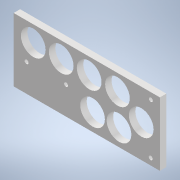
# Autodesk Inventor part: Conectores2
Saved by Autodesk Inventor 2020.3 (Build 243373000, 373)
## iProperties
Created: 2021-04-09
Part Number: Conectores2
Material: Generic
Document SubType Name: Modeling
Designer: juanp
Density: 1 g/cm^3
Appearance: Default
Autodesk Inventor part; units mm, degrees
(part 1 of 2)
ref_plane "YZ Plane" through (0, 0, 0) normal (1, 0, 0) x (0, 1, 0)
ref_plane "XZ Plane" through (0, 0, 0) normal (0, 1, 0) x (-1, 0, 0)
ref_plane "XY Plane" through (0, 0, 0) normal (0, 0, 1) x (1, 0, 0)
sketch "20" plane through (0, 0, 0) normal (0, 0, 1) x (1, 0, 0)
  line L0 (0, 0) -> (106.66, 0)
  line L1 (106.66, 0) -> (106.66, 46.914)
  line L2 (106.66, 46.914) -> (0, 46.914)
  line L3 (0, 46.914) -> (0, 0)
  arc A0 (-5.7307, 23.3678) -> (-5.7307, 23.444) centre (-5.7307, 23.4059) ccw
  line L4 (-5.821, 23.4059) -> (-5.821, 23.4962)
  arc A1 (-5.7829, 23.4962) -> (-5.8591, 23.4962) centre (-5.821, 23.4962) ccw
  arc A2 (-5.8591, 23.4059) -> (-5.7829, 23.4059) centre (-5.821, 23.4059) ccw
  line L5 (-5.821, 23.4962) -> (-5.7307, 23.4962)
  arc A3 (-5.7307, 23.4581) -> (-5.7307, 23.5343) centre (-5.7307, 23.4962) ccw
  arc A4 (-5.821, 23.5343) -> (-5.821, 23.4581) centre (-5.821, 23.4962) ccw
  line L6 (-5.7307, 23.4962) -> (-5.7307, 23.4059)
  arc A5 (-5.7688, 23.4059) -> (-5.6926, 23.4059) centre (-5.7307, 23.4059) ccw
  arc A6 (-5.6926, 23.4962) -> (-5.7688, 23.4962) centre (-5.7307, 23.4962) ccw
  line L7 (-6.4532, 24.9968) -> (-6.4532, 24.4549)
  arc A7 (-6.4913, 24.4549) -> (-6.4151, 24.4549) centre (-6.4532, 24.4549) ccw
  arc A8 (-6.4151, 24.9968) -> (-6.4913, 24.9968) centre (-6.4532, 24.9968) ccw
  arc A9 (-6.8144, 24.0937) -> (-6.4532, 24.4549) centre (-6.8144, 24.4549) ccw
  arc A10 (-6.8144, 24.1318) -> (-6.8144, 24.0556) centre (-6.8144, 24.0937) ccw
  arc A11 (-6.4151, 24.4549) -> (-6.4913, 24.4549) centre (-6.4532, 24.4549) ccw
  line L8 (-6.8144, 24.0937) -> (-6.9047, 24.0937)
  arc A12 (-6.9047, 24.1318) -> (-6.9047, 24.0556) centre (-6.9047, 24.0937) ccw
  arc A13 (-6.8144, 24.0556) -> (-6.8144, 24.1318) centre (-6.8144, 24.0937) ccw
  arc A14 (-6.9047, 24.9968) -> (-6.9047, 24.0937) centre (-6.9047, 24.5453) ccw
  arc A15 (-6.9047, 24.9587) -> (-6.9047, 25.0349) centre (-6.9047, 24.9968) ccw
  arc A16 (-6.9047, 24.0556) -> (-6.9047, 24.1318) centre (-6.9047, 24.0937) ccw
  line L9 (-6.9047, 24.9968) -> (-6.4532, 24.9968)
  arc A17 (-6.4532, 24.9587) -> (-6.4532, 25.0349) centre (-6.4532, 24.9968) ccw
  arc A18 (-6.9047, 25.0349) -> (-6.9047, 24.9587) centre (-6.9047, 24.9968) ccw
  arc A19 (-5.7307, 24.2743) -> (-6.4532, 24.9968) centre (-6.4532, 24.2743) ccw
  arc A20 (-5.7688, 24.2743) -> (-5.6926, 24.2743) centre (-5.7307, 24.2743) ccw
  arc A21 (-6.4532, 25.0349) -> (-6.4532, 24.9587) centre (-6.4532, 24.9968) ccw
  line L10 (-6.9951, 25.6568) -> (-7.3563, 26.1084)
  arc A22 (-7.3265, 26.1322) -> (-7.3861, 26.0846) centre (-7.3563, 26.1084) ccw
  arc A23 (-7.0248, 25.633) -> (-6.9653, 25.6806) centre (-6.9951, 25.6568) ccw
  line L11 (-7.3563, 26.1084) -> (-5.7307, 26.1084)
  arc A24 (-5.7307, 26.0703) -> (-5.7307, 26.1465) centre (-5.7307, 26.1084) ccw
  arc A25 (-7.3563, 26.1465) -> (-7.3563, 26.0703) centre (-7.3563, 26.1084) ccw
  line L12 (-5.7307, 25.6568) -> (-5.7307, 26.5599)
  arc A26 (-5.6926, 26.5599) -> (-5.7688, 26.5599) centre (-5.7307, 26.5599) ccw
  arc A27 (-5.7688, 25.6568) -> (-5.6926, 25.6568) centre (-5.7307, 25.6568) ccw
  line L13 (106.66, 46.914) -> (106.66, 51.48)
  arc A28 (106.6925, 51.48) -> (106.6275, 51.48) centre (106.66, 51.48) ccw
  arc A29 (106.6275, 46.914) -> (106.6925, 46.914) centre (106.66, 46.914) ccw
  line L14 (0, 46.914) -> (0, 51.48)
  arc A30 (0.0325, 51.48) -> (-0.0325, 51.48) centre (0, 51.48) ccw
  arc A31 (-0.0325, 46.914) -> (0.0325, 46.914) centre (0, 46.914) ccw
  line L15 (106.595, 49.53) -> (0.065, 49.53)
  arc A32 (0.065, 49.5625) -> (0.065, 49.4975) centre (0.065, 49.53) ccw
  arc A33 (106.595, 49.4975) -> (106.595, 49.5625) centre (106.595, 49.53) ccw
  line L16 (106.595, 49.53) -> (104.06, 49.8492)
  arc A34 (104.0641, 49.8815) -> (104.0559, 49.817) centre (104.06, 49.8493) ccw
  arc A35 (106.5909, 49.4978) -> (106.5991, 49.5622) centre (106.595, 49.53) ccw
  line L17 (104.06, 49.8492) -> (104.06, 49.2108)
  arc A36 (104.0275, 49.2108) -> (104.0925, 49.2108) centre (104.06, 49.2108) ccw
  arc A37 (104.0925, 49.8492) -> (104.0275, 49.8492) centre (104.06, 49.8492) ccw
  line L18 (104.06, 49.2108) -> (106.595, 49.53)
  arc A38 (106.5991, 49.4978) -> (106.5909, 49.5622) centre (106.595, 49.53) ccw
  arc A39 (104.0559, 49.243) -> (104.0641, 49.1785) centre (104.06, 49.2107) ccw
  line L19 (106.595, 49.53) -> (104.06, 49.66)
  arc A40 (104.0617, 49.6925) -> (104.0583, 49.6275) centre (104.06, 49.66) ccw
  arc A41 (106.5933, 49.4975) -> (106.5967, 49.5625) centre (106.595, 49.53) ccw
  line L20 (104.06, 49.4) -> (106.595, 49.53)
  arc A42 (106.5967, 49.4975) -> (106.5933, 49.5625) centre (106.595, 49.53) ccw
  arc A43 (104.0583, 49.4325) -> (104.0617, 49.3675) centre (104.06, 49.4) ccw
  line L21 (106.595, 49.53) -> (104.06, 49.79)
  arc A44 (104.0633, 49.8223) -> (104.0567, 49.7577) centre (104.06, 49.79) ccw
  arc A45 (106.5917, 49.4977) -> (106.5983, 49.5623) centre (106.595, 49.53) ccw
  line L22 (104.06, 49.27) -> (106.595, 49.53)
  arc A46 (106.5983, 49.4977) -> (106.5917, 49.5623) centre (106.595, 49.53) ccw
  arc A47 (104.0567, 49.3023) -> (104.0633, 49.2377) centre (104.06, 49.27) ccw
  line L23 (0.065, 49.53) -> (2.6, 49.8492)
  arc A48 (2.6041, 49.817) -> (2.5959, 49.8815) centre (2.6, 49.8493) ccw
  arc A49 (0.0609, 49.5622) -> (0.0691, 49.4978) centre (0.065, 49.53) ccw
  line L24 (2.6, 49.8492) -> (2.6, 49.2108)
  arc A50 (2.5675, 49.2108) -> (2.6325, 49.2108) centre (2.6, 49.2108) ccw
  arc A51 (2.6325, 49.8492) -> (2.5675, 49.8492) centre (2.6, 49.8492) ccw
  line L25 (2.6, 49.2108) -> (0.065, 49.53)
  arc A52 (0.0691, 49.5622) -> (0.0609, 49.4978) centre (0.065, 49.53) ccw
  arc A53 (2.5959, 49.1785) -> (2.6041, 49.243) centre (2.6, 49.2107) ccw
  line L26 (0.065, 49.53) -> (2.6, 49.66)
  arc A54 (2.6017, 49.6275) -> (2.5983, 49.6925) centre (2.6, 49.66) ccw
  arc A55 (0.0633, 49.5625) -> (0.0667, 49.4975) centre (0.065, 49.53) ccw
  line L27 (2.6, 49.4) -> (0.065, 49.53)
  arc A56 (0.0667, 49.5625) -> (0.0633, 49.4975) centre (0.065, 49.53) ccw
  arc A57 (2.5983, 49.3675) -> (2.6017, 49.4325) centre (2.6, 49.4) ccw
  line L28 (0.065, 49.53) -> (2.6, 49.79)
  arc A58 (2.6033, 49.7577) -> (2.5967, 49.8223) centre (2.6, 49.79) ccw
  arc A59 (0.0617, 49.5623) -> (0.0683, 49.4977) centre (0.065, 49.53) ccw
  line L29 (2.6, 49.27) -> (0.065, 49.53)
  arc A60 (0.0683, 49.5623) -> (0.0617, 49.4977) centre (0.065, 49.53) ccw
  arc A61 (2.5967, 49.2377) -> (2.6033, 49.3023) centre (2.6, 49.27) ccw
  line L30 (49.5056, 51.4451) -> (49.9571, 51.8063)
  arc A62 (49.9809, 51.7765) -> (49.9333, 51.8361) centre (49.9571, 51.8063) ccw
  arc A63 (49.4818, 51.4748) -> (49.5294, 51.4153) centre (49.5056, 51.4451) ccw
  line L31 (49.9571, 51.8063) -> (49.9571, 50.1807)
  arc A64 (49.919, 50.1807) -> (49.9952, 50.1807) centre (49.9571, 50.1807) ccw
  arc A65 (49.9952, 51.8063) -> (49.919, 51.8063) centre (49.9571, 51.8063) ccw
  line L32 (49.5056, 50.1807) -> (50.4087, 50.1807)
  arc A66 (50.4087, 50.1426) -> (50.4087, 50.2188) centre (50.4087, 50.1807) ccw
  arc A67 (49.5056, 50.2188) -> (49.5056, 50.1426) centre (49.5056, 50.1807) ccw
  arc A68 (51.2042, 51.5805) -> (51.0687, 50.9935) centre (52.4081, 50.9934) ccw
  arc A69 (51.2384, 51.5638) -> (51.1699, 51.5972) centre (51.2042, 51.5805) ccw
  arc A70 (51.0306, 50.9935) -> (51.1068, 50.9935) centre (51.0687, 50.9935) ccw
  arc A71 (51.5203, 51.8063) -> (51.2042, 51.5805) centre (51.5203, 51.4722) ccw
  arc A72 (51.5203, 51.7682) -> (51.5203, 51.8444) centre (51.5203, 51.8063) ccw
  arc A73 (51.1681, 51.5929) -> (51.2402, 51.5682) centre (51.2042, 51.5806) ccw
  arc A74 (51.8364, 51.5805) -> (51.5203, 51.8063) centre (51.5203, 51.4722) ccw
  arc A75 (51.8003, 51.5682) -> (51.8724, 51.5929) centre (51.8363, 51.5806) ccw
  arc A76 (51.5203, 51.8444) -> (51.5203, 51.7682) centre (51.5203, 51.8063) ccw
  arc A77 (51.9718, 50.9935) -> (51.8364, 51.5805) centre (50.6324, 50.9937) ccw
  arc A78 (51.9337, 50.9935) -> (52.0099, 50.9935) centre (51.9718, 50.9935) ccw
  arc A79 (51.8706, 51.5972) -> (51.8021, 51.5638) centre (51.8364, 51.5805) ccw
  arc A80 (51.0687, 50.9935) -> (51.2042, 50.4065) centre (52.4081, 50.9936) ccw
  arc A81 (51.1068, 50.9935) -> (51.0306, 50.9935) centre (51.0687, 50.9935) ccw
  arc A82 (51.1699, 50.3898) -> (51.2384, 50.4232) centre (51.2042, 50.4065) ccw
  arc A83 (51.2042, 50.4065) -> (51.5203, 50.1807) centre (51.5203, 50.5148) ccw
  arc A84 (51.2402, 50.4188) -> (51.1681, 50.3941) centre (51.2042, 50.4065) ccw
  arc A85 (51.5203, 50.1426) -> (51.5203, 50.2188) centre (51.5203, 50.1807) ccw
  arc A86 (51.8364, 50.4065) -> (51.9718, 50.9935) centre (50.6324, 50.9933) ccw
  arc A87 (51.8021, 50.4232) -> (51.8706, 50.3898) centre (51.8364, 50.4065) ccw
  arc A88 (52.0099, 50.9935) -> (51.9337, 50.9935) centre (51.9718, 50.9935) ccw
  arc A89 (51.5203, 50.1807) -> (51.8364, 50.4065) centre (51.5203, 50.5148) ccw
  arc A90 (51.5203, 50.2188) -> (51.5203, 50.1426) centre (51.5203, 50.1807) ccw
  arc A91 (51.8724, 50.3941) -> (51.8003, 50.4188) centre (51.8363, 50.4065) ccw
  line L33 (51.159, 50.5419) -> (51.8815, 51.4451)
  arc A92 (51.9113, 51.4213) -> (51.8518, 51.4689) centre (51.8816, 51.4451) ccw
  arc A93 (51.1293, 50.5657) -> (51.1888, 50.5181) centre (51.1591, 50.5419) ccw
  line L34 (52.6318, 51.0838) -> (53.1737, 51.0838)
  arc A94 (53.1737, 51.0457) -> (53.1737, 51.1219) centre (53.1737, 51.0838) ccw
  arc A95 (52.6318, 51.1219) -> (52.6318, 51.0457) centre (52.6318, 51.0838) ccw
  arc A96 (53.5349, 50.7226) -> (53.1737, 51.0838) centre (53.1737, 50.7226) ccw
  arc A97 (53.4968, 50.7226) -> (53.573, 50.7226) centre (53.5349, 50.7226) ccw
  arc A98 (53.1737, 51.1219) -> (53.1737, 51.0457) centre (53.1737, 51.0838) ccw
  line L35 (53.5349, 50.7226) -> (53.5349, 50.6323)
  arc A99 (53.4968, 50.6323) -> (53.573, 50.6323) centre (53.5349, 50.6323) ccw
  arc A100 (53.573, 50.7226) -> (53.4968, 50.7226) centre (53.5349, 50.7226) ccw
  arc A101 (52.6318, 50.6323) -> (53.5349, 50.6323) centre (53.0833, 50.6323) ccw
  arc A102 (52.6699, 50.6323) -> (52.5937, 50.6323) centre (52.6318, 50.6323) ccw
  arc A103 (53.573, 50.6323) -> (53.4968, 50.6323) centre (53.5349, 50.6323) ccw
  line L36 (52.6318, 50.6323) -> (52.6318, 51.0838)
  arc A104 (52.6699, 51.0838) -> (52.5937, 51.0838) centre (52.6318, 51.0838) ccw
  arc A105 (56.3452, 50.6323) -> (56.4214, 50.6323) centre (56.3833, 50.6323) ccw
  arc A106 (52.5937, 50.6323) -> (52.6699, 50.6323) centre (52.6318, 50.6323) ccw
  arc A107 (53.3543, 51.8063) -> (52.6318, 51.0838) centre (53.3543, 51.0838) ccw
  arc A108 (53.3543, 51.7682) -> (53.3543, 51.8444) centre (53.3543, 51.8063) ccw
  arc A109 (52.5937, 51.0838) -> (52.6699, 51.0838) centre (52.6318, 51.0838) ccw
  line L37 (54.1324, 50.1807) -> (54.1324, 50.271)
  arc A110 (54.1705, 50.271) -> (54.0943, 50.271) centre (54.1324, 50.271) ccw
  arc A111 (54.0943, 50.1807) -> (54.1705, 50.1807) centre (54.1324, 50.1807) ccw
  line L38 (54.1324, 50.271) -> (54.2227, 50.271)
  arc A112 (54.2227, 50.2329) -> (54.2227, 50.3091) centre (54.2227, 50.271) ccw
  arc A113 (54.1324, 50.3091) -> (54.1324, 50.2329) centre (54.1324, 50.271) ccw
  line L39 (54.2227, 50.271) -> (54.2227, 50.1807)
  arc A114 (54.1846, 50.1807) -> (54.2608, 50.1807) centre (54.2227, 50.1807) ccw
  arc A115 (54.2608, 50.271) -> (54.1846, 50.271) centre (54.2227, 50.271) ccw
  line L40 (54.2227, 50.1807) -> (54.1324, 50.1807)
  arc A116 (54.1324, 50.2188) -> (54.1324, 50.1426) centre (54.1324, 50.1807) ccw
  arc A117 (54.2227, 50.1426) -> (54.2227, 50.2188) centre (54.2227, 50.1807) ccw
  arc A118 (55.3621, 51.0457) -> (55.3621, 51.1219) centre (55.3621, 51.0838) ccw
  arc A119 (54.8202, 51.1219) -> (54.8202, 51.0457) centre (54.8202, 51.0838) ccw
  arc A120 (55.7233, 50.7226) -> (55.3621, 51.0838) centre (55.3621, 50.7226) ccw
  arc A121 (55.6852, 50.7226) -> (55.7614, 50.7226) centre (55.7233, 50.7226) ccw
  arc A122 (55.3621, 51.1219) -> (55.3621, 51.0457) centre (55.3621, 51.0838) ccw
  line L41 (55.7233, 50.7226) -> (55.7233, 50.6323)
  arc A123 (55.6852, 50.6323) -> (55.7614, 50.6323) centre (55.7233, 50.6323) ccw
  arc A124 (55.7614, 50.7226) -> (55.6852, 50.7226) centre (55.7233, 50.7226) ccw
  arc A125 (54.8202, 50.6323) -> (55.7233, 50.6323) centre (55.2717, 50.6323) ccw
  arc A126 (54.8583, 50.6323) -> (54.7821, 50.6323) centre (54.8202, 50.6323) ccw
  arc A127 (55.7614, 50.6323) -> (55.6852, 50.6323) centre (55.7233, 50.6323) ccw
  line L42 (54.8202, 50.6323) -> (54.8202, 51.0838)
  arc A128 (54.8583, 51.0838) -> (54.7821, 51.0838) centre (54.8202, 51.0838) ccw
  arc A129 (54.7821, 50.6323) -> (54.8583, 50.6323) centre (54.8202, 50.6323) ccw
  arc A130 (55.5427, 51.8063) -> (54.8202, 51.0838) centre (55.5427, 51.0838) ccw
  arc A131 (55.5427, 51.7682) -> (55.5427, 51.8444) centre (55.5427, 51.8063) ccw
  arc A132 (54.7821, 51.0838) -> (54.8583, 51.0838) centre (54.8202, 51.0838) ccw
  line L43 (56.3833, 51.0838) -> (56.9252, 51.0838)
  arc A133 (56.9252, 51.0457) -> (56.9252, 51.1219) centre (56.9252, 51.0838) ccw
  arc A134 (56.3833, 51.1219) -> (56.3833, 51.0457) centre (56.3833, 51.0838) ccw
  arc A135 (57.2864, 50.7226) -> (56.9252, 51.0838) centre (56.9252, 50.7226) ccw
  arc A136 (57.2483, 50.7226) -> (57.3245, 50.7226) centre (57.2864, 50.7226) ccw
  arc A137 (56.9252, 51.1219) -> (56.9252, 51.0457) centre (56.9252, 51.0838) ccw
  line L44 (57.2864, 50.7226) -> (57.2864, 50.6323)
  arc A138 (57.2483, 50.6323) -> (57.3245, 50.6323) centre (57.2864, 50.6323) ccw
  arc A139 (57.3245, 50.7226) -> (57.2483, 50.7226) centre (57.2864, 50.7226) ccw
  arc A140 (56.3833, 50.6323) -> (57.2864, 50.6323) centre (56.8349, 50.6323) ccw
  arc A141 (56.4214, 50.6323) -> (56.3452, 50.6323) centre (56.3833, 50.6323) ccw
  arc A142 (57.3245, 50.6323) -> (57.2483, 50.6323) centre (57.2864, 50.6323) ccw
  line L45 (56.3833, 50.6323) -> (56.3833, 51.0838)
  arc A143 (56.4214, 51.0838) -> (56.3452, 51.0838) centre (56.3833, 51.0838) ccw
  line L46 (2.54, 46.914) -> (-7.03, 46.914)
  arc A144 (-7.03, 46.9465) -> (-7.03, 46.8815) centre (-7.03, 46.914) ccw
  arc A145 (2.54, 46.8815) -> (2.54, 46.9465) centre (2.54, 46.914) ccw
  line L47 (2.54, 0) -> (-7.03, 0)
  arc A146 (-7.03, 0.0325) -> (-7.03, -0.0325) centre (-7.03, 0) ccw
  arc A147 (2.54, -0.0325) -> (2.54, 0.0325) centre (2.54, 0) ccw
  line L48 (-5.08, 46.849) -> (-5.08, 0.065)
  arc A148 (-5.1125, 0.065) -> (-5.0475, 0.065) centre (-5.08, 0.065) ccw
  arc A149 (-5.0475, 46.849) -> (-5.1125, 46.849) centre (-5.08, 46.849) ccw
  line L49 (-5.08, 46.849) -> (-5.3992, 44.314)
  arc A150 (-5.4315, 44.3181) -> (-5.367, 44.3099) centre (-5.3993, 44.314) ccw
  arc A151 (-5.0478, 46.8449) -> (-5.1122, 46.8531) centre (-5.08, 46.849) ccw
  line L50 (-5.3992, 44.314) -> (-4.7608, 44.314)
  arc A152 (-4.7608, 44.2815) -> (-4.7608, 44.3465) centre (-4.7608, 44.314) ccw
  arc A153 (-5.3992, 44.3465) -> (-5.3992, 44.2815) centre (-5.3992, 44.314) ccw
  line L51 (-4.7608, 44.314) -> (-5.08, 46.849)
  arc A154 (-5.0478, 46.8531) -> (-5.1122, 46.8449) centre (-5.08, 46.849) ccw
  arc A155 (-4.793, 44.3099) -> (-4.7285, 44.3181) centre (-4.7607, 44.314) ccw
  line L52 (-5.08, 46.849) -> (-5.21, 44.314)
  arc A156 (-5.2425, 44.3157) -> (-5.1775, 44.3123) centre (-5.21, 44.314) ccw
  arc A157 (-5.0475, 46.8473) -> (-5.1125, 46.8507) centre (-5.08, 46.849) ccw
  line L53 (-4.95, 44.314) -> (-5.08, 46.849)
  arc A158 (-5.0475, 46.8507) -> (-5.1125, 46.8473) centre (-5.08, 46.849) ccw
  arc A159 (-4.9825, 44.3123) -> (-4.9175, 44.3157) centre (-4.95, 44.314) ccw
  line L54 (-5.08, 46.849) -> (-5.34, 44.314)
  arc A160 (-5.3723, 44.3173) -> (-5.3077, 44.3107) centre (-5.34, 44.314) ccw
  arc A161 (-5.0477, 46.8457) -> (-5.1123, 46.8523) centre (-5.08, 46.849) ccw
  line L55 (-4.82, 44.314) -> (-5.08, 46.849)
  arc A162 (-5.0477, 46.8523) -> (-5.1123, 46.8457) centre (-5.08, 46.849) ccw
  arc A163 (-4.8523, 44.3107) -> (-4.7877, 44.3173) centre (-4.82, 44.314) ccw
  line L56 (-5.08, 0.065) -> (-5.3992, 2.6)
  arc A164 (-5.367, 2.6041) -> (-5.4315, 2.5959) centre (-5.3993, 2.6) ccw
  arc A165 (-5.1122, 0.0609) -> (-5.0478, 0.0691) centre (-5.08, 0.065) ccw
  line L57 (-5.3992, 2.6) -> (-4.7608, 2.6)
  arc A166 (-4.7608, 2.5675) -> (-4.7608, 2.6325) centre (-4.7608, 2.6) ccw
  arc A167 (-5.3992, 2.6325) -> (-5.3992, 2.5675) centre (-5.3992, 2.6) ccw
  line L58 (-4.7608, 2.6) -> (-5.08, 0.065)
  arc A168 (-5.1122, 0.0691) -> (-5.0478, 0.0609) centre (-5.08, 0.065) ccw
  arc A169 (-4.7285, 2.5959) -> (-4.793, 2.6041) centre (-4.7607, 2.6) ccw
  line L59 (-5.08, 0.065) -> (-5.21, 2.6)
  arc A170 (-5.1775, 2.6017) -> (-5.2425, 2.5983) centre (-5.21, 2.6) ccw
  arc A171 (-5.1125, 0.0633) -> (-5.0475, 0.0667) centre (-5.08, 0.065) ccw
  line L60 (-4.95, 2.6) -> (-5.08, 0.065)
  arc A172 (-5.1125, 0.0667) -> (-5.0475, 0.0633) centre (-5.08, 0.065) ccw
  arc A173 (-4.9175, 2.5983) -> (-4.9825, 2.6017) centre (-4.95, 2.6) ccw
  line L61 (-5.08, 0.065) -> (-5.34, 2.6)
  arc A174 (-5.3077, 2.6033) -> (-5.3723, 2.5967) centre (-5.34, 2.6) ccw
  arc A175 (-5.1123, 0.0617) -> (-5.0477, 0.0683) centre (-5.08, 0.065) ccw
  line L62 (-4.82, 2.6) -> (-5.08, 0.065)
  arc A176 (-5.1123, 0.0683) -> (-5.0477, 0.0617) centre (-5.08, 0.065) ccw
  arc A177 (-4.7877, 2.5967) -> (-4.8523, 2.6033) centre (-4.82, 2.6) ccw
  line L63 (-7.3563, 20.7034) -> (-6.0919, 20.3422)
  arc A178 (-6.1024, 20.3056) -> (-6.0815, 20.3788) centre (-6.092, 20.3422) ccw
  arc A179 (-7.3458, 20.7401) -> (-7.3668, 20.6668) centre (-7.3563, 20.7035) ccw
  line L64 (-6.0919, 20.3422) -> (-6.0919, 21.2453)
  arc A180 (-6.0538, 21.2453) -> (-6.13, 21.2453) centre (-6.0919, 21.2453) ccw
  arc A181 (-6.13, 20.3422) -> (-6.0538, 20.3422) centre (-6.0919, 20.3422) ccw
  line L65 (-6.4532, 20.9744) -> (-5.7307, 20.9744)
  arc A182 (-5.7307, 20.9363) -> (-5.7307, 21.0125) centre (-5.7307, 20.9744) ccw
  arc A183 (-6.4532, 21.0125) -> (-6.4532, 20.9363) centre (-6.4532, 20.9744) ccw
  line L66 (-6.6338, 21.9053) -> (-6.6338, 22.4472)
  arc A184 (-6.5957, 22.4472) -> (-6.6719, 22.4472) centre (-6.6338, 22.4472) ccw
  arc A185 (-6.6719, 21.9053) -> (-6.5957, 21.9053) centre (-6.6338, 21.9053) ccw
  arc A186 (-6.2726, 22.8084) -> (-6.6338, 22.4472) centre (-6.2726, 22.4472) ccw
  arc A187 (-6.2726, 22.7703) -> (-6.2726, 22.8465) centre (-6.2726, 22.8084) ccw
  arc A188 (-6.6719, 22.4472) -> (-6.5957, 22.4472) centre (-6.6338, 22.4472) ccw
  line L67 (-6.2726, 22.8084) -> (-6.1823, 22.8084)
  arc A189 (-6.1823, 22.7703) -> (-6.1823, 22.8465) centre (-6.1823, 22.8084) ccw
  arc A190 (-6.2726, 22.8465) -> (-6.2726, 22.7703) centre (-6.2726, 22.8084) ccw
  arc A191 (-6.1823, 21.9053) -> (-6.1823, 22.8084) centre (-6.1823, 22.3569) ccw
  arc A192 (-6.1823, 21.9434) -> (-6.1823, 21.8672) centre (-6.1823, 21.9053) ccw
  arc A193 (-6.1823, 22.8465) -> (-6.1823, 22.7703) centre (-6.1823, 22.8084) ccw
  line L68 (-6.1823, 21.9053) -> (-6.6338, 21.9053)
  arc A194 (-6.6338, 21.9434) -> (-6.6338, 21.8672) centre (-6.6338, 21.9053) ccw
  arc A195 (-6.1823, 21.8672) -> (-6.1823, 21.9434) centre (-6.1823, 21.9053) ccw
  arc A196 (-7.3563, 22.6278) -> (-6.6338, 21.9053) centre (-6.6338, 22.6278) ccw
  arc A197 (-7.3182, 22.6278) -> (-7.3944, 22.6278) centre (-7.3563, 22.6278) ccw
  arc A198 (-6.6338, 21.8672) -> (-6.6338, 21.9434) centre (-6.6338, 21.9053) ccw
  line L69 (-5.7307, 23.4059) -> (-5.821, 23.4059)
  arc A199 (-5.821, 23.444) -> (-5.821, 23.3678) centre (-5.821, 23.4059) ccw
  arc A200 (57.1058, 51.8063) -> (56.3833, 51.0838) centre (57.1058, 51.0838) ccw
  arc A201 (57.1058, 51.7682) -> (57.1058, 51.8444) centre (57.1058, 51.8063) ccw
  arc A202 (56.3452, 51.0838) -> (56.4214, 51.0838) centre (56.3833, 51.0838) ccw
  circle A203 centre (6.998, 20.3594) radius 1.51
  circle A204 centre (37.3779, 20.3594) radius 1.51
  circle A205 centre (102.615, 42.9184) radius 1.51
  circle A206 centre (102.502, 4.0549) radius 1.51
  line L70 (54.8202, 51.0838) -> (55.3621, 51.0838)
  constraints: 501 point on circle, 207 centre point, 142 end point, 56 point on line
sketch "21" plane through (0, 0, 0) normal (0, 0, 1) x (1, 0, 0)
  line L0 (56.8302, 12.0686) -> (57.1435, 12.0686)
  line L1 (2.5931, 11.0351) -> (22.5931, 11.0351)
  arc A0 (22.5931, 10.9843) -> (22.5931, 11.0859) centre (22.5931, 11.0351) ccw
  arc A1 (2.5931, 11.0859) -> (2.5931, 10.9843) centre (2.5931, 11.0351) ccw
  line L2 (22.5931, 11.0351) -> (22.5931, 2.6351)
  arc A2 (22.5423, 2.6351) -> (22.6439, 2.6351) centre (22.5931, 2.6351) ccw
  arc A3 (22.6439, 11.0351) -> (22.5423, 11.0351) centre (22.5931, 11.0351) ccw
  line L3 (22.5931, 2.6351) -> (18.5311, 2.6351)
  arc A4 (18.5311, 2.6859) -> (18.5311, 2.5843) centre (18.5311, 2.6351) ccw
  arc A5 (22.5931, 2.5843) -> (22.5931, 2.6859) centre (22.5931, 2.6351) ccw
  line L4 (18.5311, 2.6351) -> (18.5311, 2.9351)
  arc A6 (18.5819, 2.9351) -> (18.4803, 2.9351) centre (18.5311, 2.9351) ccw
  arc A7 (18.4803, 2.6351) -> (18.5819, 2.6351) centre (18.5311, 2.6351) ccw
  line L5 (18.5311, 2.9351) -> (17.0521, 2.9351)
  arc A8 (17.0521, 2.9859) -> (17.0521, 2.8843) centre (17.0521, 2.9351) ccw
  arc A9 (18.5311, 2.8843) -> (18.5311, 2.9859) centre (18.5311, 2.9351) ccw
  line L6 (17.0521, 2.9351) -> (17.0521, 2.6351)
  arc A10 (17.0013, 2.6351) -> (17.1029, 2.6351) centre (17.0521, 2.6351) ccw
  arc A11 (17.1029, 2.9351) -> (17.0013, 2.9351) centre (17.0521, 2.9351) ccw
  line L7 (17.0521, 2.6351) -> (14.4761, 2.6351)
  arc A12 (14.4761, 2.6859) -> (14.4761, 2.5843) centre (14.4761, 2.6351) ccw
  arc A13 (17.0521, 2.5843) -> (17.0521, 2.6859) centre (17.0521, 2.6351) ccw
  line L8 (14.4761, 2.6351) -> (14.4761, 4.1851)
  arc A14 (14.5269, 4.1851) -> (14.4253, 4.1851) centre (14.4761, 4.1851) ccw
  arc A15 (14.4253, 2.6351) -> (14.5269, 2.6351) centre (14.4761, 2.6351) ccw
  line L9 (14.4761, 4.1851) -> (10.7101, 4.1851)
  arc A16 (10.7101, 4.2359) -> (10.7101, 4.1343) centre (10.7101, 4.1851) ccw
  arc A17 (14.4761, 4.1343) -> (14.4761, 4.2359) centre (14.4761, 4.1851) ccw
  line L10 (10.7101, 4.1851) -> (10.7101, 2.6351)
  arc A18 (10.6593, 2.6351) -> (10.7609, 2.6351) centre (10.7101, 2.6351) ccw
  arc A19 (10.7609, 4.1851) -> (10.6593, 4.1851) centre (10.7101, 4.1851) ccw
  line L11 (14.4761, 2.6351) -> (10.7101, 2.6351)
  arc A20 (10.7101, 2.6859) -> (10.7101, 2.5843) centre (10.7101, 2.6351) ccw
  arc A21 (76.2324, 34.6718) -> (76.2324, 34.6337) centre (76.2324, 34.6527) ccw
  arc A22 (76.2324, 35.1939) -> (76.2324, 35.1558) centre (76.2324, 35.1748) ccw
  line L12 (75.9714, 35.5925) -> (76.2847, 35.5925)
  arc A23 (76.2847, 35.5735) -> (76.2847, 35.6116) centre (76.2847, 35.5926) ccw
  arc A24 (75.9714, 35.6116) -> (75.9714, 35.5735) centre (75.9714, 35.5926) ccw
  arc A25 (76.2847, 35.1748) -> (76.2847, 35.5925) centre (76.2847, 35.3837) ccw
  arc A26 (76.2847, 35.1939) -> (76.2847, 35.1558) centre (76.2847, 35.1748) ccw
  arc A27 (76.2847, 35.6116) -> (76.2847, 35.5735) centre (76.2847, 35.5926) ccw
  line L13 (76.2847, 35.1748) -> (76.0758, 35.1748)
  arc A28 (76.0758, 35.1939) -> (76.0758, 35.1558) centre (76.0758, 35.1748) ccw
  arc A29 (75.9714, 34.6718) -> (75.9714, 34.6337) centre (75.9714, 34.6527) ccw
  arc A30 (76.9333, 27.6146) -> (76.9333, 43.6146) centre (76.9333, 35.6146) ccw
  arc A31 (76.9333, 43.6146) -> (76.9333, 27.6146) centre (76.9333, 35.6146) ccw
  arc A32 (76.9333, 29.0954) -> (76.9333, 42.1338) centre (76.9333, 35.6146) ccw
  arc A33 (76.9333, 42.1338) -> (76.9333, 29.0954) centre (76.9333, 35.6146) ccw
  arc A34 (76.9333, 26.1146) -> (76.9333, 45.1146) centre (76.9333, 35.6146) ccw
  arc A35 (76.9333, 45.1146) -> (76.9333, 26.1146) centre (76.9333, 35.6146) ccw
  arc A36 (2.6439, 11.0351) -> (2.5423, 11.0351) centre (2.5931, 11.0351) ccw
  arc A37 (58.7921, 5.5907) -> (56.7921, 5.5907) centre (57.7921, 5.5907) ccw
  arc A38 (58.7604, 5.5907) -> (58.8239, 5.5907) centre (58.7922, 5.5907) ccw
  arc A39 (56.7604, 5.5907) -> (56.8239, 5.5907) centre (56.7921, 5.5907) ccw
  line L14 (62.8302, 11.8597) -> (63.0913, 12.0686)
  arc A40 (63.1032, 12.0537) -> (63.0794, 12.0834) centre (63.0913, 12.0686) ccw
  arc A41 (62.8183, 11.8746) -> (62.8421, 11.8448) centre (62.8302, 11.8597) ccw
  line L15 (63.0913, 12.0686) -> (63.0913, 11.1288)
  arc A42 (63.0722, 11.1288) -> (63.1103, 11.1288) centre (63.0913, 11.1288) ccw
  arc A43 (63.1103, 12.0686) -> (63.0722, 12.0686) centre (63.0913, 12.0686) ccw
  line L16 (62.8302, 11.1288) -> (63.3523, 11.1288)
  arc A44 (63.3523, 11.1097) -> (63.3523, 11.1478) centre (63.3523, 11.1288) ccw
  arc A45 (62.8302, 11.1478) -> (62.8302, 11.1097) centre (62.8302, 11.1288) ccw
  arc A46 (60.3523, 16.8336) -> (60.1174, 17.0686) centre (60.1173, 16.8336) ccw
  arc A47 (60.3333, 16.8336) -> (60.3714, 16.8336) centre (60.3524, 16.8336) ccw
  arc A48 (60.1174, 17.0876) -> (60.1174, 17.0495) centre (60.1174, 17.0686) ccw
  arc A49 (60.1174, 17.0686) -> (59.8302, 16.8597) centre (60.1174, 16.7667) ccw
  arc A50 (60.1174, 17.0495) -> (60.1174, 17.0876) centre (60.1174, 17.0686) ccw
  arc A51 (59.8121, 16.8656) -> (59.8483, 16.8538) centre (59.8302, 16.8597) ccw
  arc A52 (60.274, 16.6509) -> (60.3523, 16.8336) centre (60.0999, 16.8336) ccw
  arc A53 (60.2609, 16.6647) -> (60.2871, 16.6371) centre (60.274, 16.6509) ccw
  arc A54 (60.3714, 16.8336) -> (60.3333, 16.8336) centre (60.3524, 16.8336) ccw
  line L17 (60.274, 16.6509) -> (59.8302, 16.1288)
  arc A55 (59.8157, 16.1411) -> (59.8447, 16.1164) centre (59.8302, 16.1288) ccw
  arc A56 (60.2885, 16.6385) -> (60.2595, 16.6632) centre (60.274, 16.6508) ccw
  line L18 (59.8302, 16.1288) -> (60.3523, 16.1288)
  arc A57 (60.3523, 16.1097) -> (60.3523, 16.1478) centre (60.3523, 16.1288) ccw
  arc A58 (59.8302, 16.1478) -> (59.8302, 16.1097) centre (59.8302, 16.1288) ccw
  line L19 (56.8302, 11.1288) -> (57.0913, 11.1288)
  arc A59 (57.0913, 11.1097) -> (57.0913, 11.1478) centre (57.0913, 11.1288) ccw
  arc A60 (56.8302, 11.1478) -> (56.8302, 11.1097) centre (56.8302, 11.1288) ccw
  arc A61 (57.0913, 11.1288) -> (57.0913, 11.6509) centre (57.0913, 11.3898) ccw
  arc A62 (57.0913, 11.1478) -> (57.0913, 11.1097) centre (57.0913, 11.1288) ccw
  arc A63 (57.0913, 11.6699) -> (57.0913, 11.6318) centre (57.0913, 11.6509) ccw
  arc A64 (80.6119, 16.6647) -> (80.6381, 16.6371) centre (80.625, 16.6509) ccw
  arc A65 (57.1435, 12.0495) -> (57.1435, 12.0876) centre (57.1435, 12.0686) ccw
  arc A66 (56.8302, 12.0876) -> (56.8302, 12.0495) centre (56.8302, 12.0686) ccw
  arc A67 (57.1435, 11.6509) -> (57.1435, 12.0686) centre (57.1435, 11.8598) ccw
  arc A68 (57.1435, 11.6699) -> (57.1435, 11.6318) centre (57.1435, 11.6509) ccw
  arc A69 (57.1435, 12.0876) -> (57.1435, 12.0495) centre (57.1435, 12.0686) ccw
  line L20 (57.1435, 11.6509) -> (56.9346, 11.6509)
  arc A70 (56.9346, 11.6699) -> (56.9346, 11.6318) centre (56.9346, 11.6509) ccw
  arc A71 (57.1435, 11.6318) -> (57.1435, 11.6699) centre (57.1435, 11.6509) ccw
  arc A72 (57.7921, 4.0907) -> (57.7921, 20.0907) centre (57.7921, 12.0907) ccw
  arc A73 (57.7921, 20.0907) -> (57.7921, 4.0907) centre (57.7921, 12.0907) ccw
  arc A74 (57.7921, 5.5715) -> (57.7921, 18.6099) centre (57.7921, 12.0907) ccw
  arc A75 (57.7921, 18.6099) -> (57.7921, 5.5715) centre (57.7921, 12.0907) ccw
  arc A76 (57.7921, 2.5907) -> (57.7921, 21.5907) centre (57.7921, 12.0907) ccw
  arc A77 (57.7921, 21.5907) -> (57.7921, 2.5907) centre (57.7921, 12.0907) ccw
  line L21 (2.5931, 2.6351) -> (2.5931, 11.0351)
  arc A78 (56.174, 29.1146) -> (54.174, 29.1146) centre (55.174, 29.1146) ccw
  arc A79 (56.1422, 29.1146) -> (56.2057, 29.1146) centre (56.174, 29.1146) ccw
  arc A80 (54.1422, 29.1146) -> (54.2057, 29.1146) centre (54.174, 29.1146) ccw
  line L22 (60.2121, 35.3837) -> (60.4731, 35.5925)
  arc A81 (60.485, 35.5776) -> (60.4612, 35.6074) centre (60.4731, 35.5925) ccw
  arc A82 (60.2002, 35.3985) -> (60.224, 35.3688) centre (60.2121, 35.3837) ccw
  line L23 (60.4731, 35.5925) -> (60.4731, 34.6527)
  arc A83 (60.4541, 34.6527) -> (60.4922, 34.6527) centre (60.4732, 34.6527) ccw
  arc A84 (60.4922, 35.5925) -> (60.4541, 35.5925) centre (60.4732, 35.5925) ccw
  line L24 (60.2121, 34.6527) -> (60.7342, 34.6527)
  arc A85 (60.7342, 34.6337) -> (60.7342, 34.6718) centre (60.7342, 34.6527) ccw
  arc A86 (60.2121, 34.6718) -> (60.2121, 34.6337) centre (60.2121, 34.6527) ccw
  arc A87 (57.7342, 40.3576) -> (57.4992, 40.5925) centre (57.4992, 40.3575) ccw
  arc A88 (57.7151, 40.3576) -> (57.7532, 40.3576) centre (57.7341, 40.3576) ccw
  arc A89 (57.4992, 40.6116) -> (57.4992, 40.5735) centre (57.4992, 40.5926) ccw
  arc A90 (57.4992, 40.5925) -> (57.2121, 40.3837) centre (57.4992, 40.2907) ccw
  arc A91 (57.4992, 40.5735) -> (57.4992, 40.6116) centre (57.4992, 40.5926) ccw
  arc A92 (57.1939, 40.3895) -> (57.2302, 40.3778) centre (57.2121, 40.3837) ccw
  arc A93 (57.6559, 40.1748) -> (57.7342, 40.3576) centre (57.4817, 40.3576) ccw
  arc A94 (57.6427, 40.1886) -> (57.669, 40.161) centre (57.6559, 40.1748) ccw
  arc A95 (57.7532, 40.3576) -> (57.7151, 40.3576) centre (57.7341, 40.3576) ccw
  line L25 (57.6559, 40.1748) -> (57.2121, 39.6527)
  arc A96 (57.1975, 39.665) -> (57.2266, 39.6404) centre (57.2121, 39.6527) ccw
  arc A97 (57.6704, 40.1625) -> (57.6413, 40.1872) centre (57.6559, 40.1748) ccw
  line L26 (57.2121, 39.6527) -> (57.7342, 39.6527)
  arc A98 (57.7342, 39.6337) -> (57.7342, 39.6718) centre (57.7342, 39.6527) ccw
  arc A99 (57.2121, 39.6718) -> (57.2121, 39.6337) centre (57.2121, 39.6528) ccw
  line L27 (54.2121, 34.6527) -> (54.4731, 34.6527)
  arc A100 (54.4731, 34.6337) -> (54.4731, 34.6718) centre (54.4731, 34.6527) ccw
  arc A101 (54.2121, 34.6718) -> (54.2121, 34.6337) centre (54.2121, 34.6527) ccw
  arc A102 (54.4731, 34.6527) -> (54.4731, 35.1748) centre (54.4731, 34.9138) ccw
  arc A103 (54.4731, 34.6718) -> (54.4731, 34.6337) centre (54.4731, 34.6527) ccw
  arc A104 (54.4731, 35.1939) -> (54.4731, 35.1558) centre (54.4731, 35.1748) ccw
  line L28 (54.2121, 35.5925) -> (54.5253, 35.5925)
  arc A105 (54.5253, 35.5735) -> (54.5253, 35.6116) centre (54.5253, 35.5926) ccw
  arc A106 (54.2121, 35.6116) -> (54.2121, 35.5735) centre (54.2121, 35.5926) ccw
  arc A107 (54.5253, 35.1748) -> (54.5253, 35.5925) centre (54.5253, 35.3837) ccw
  arc A108 (54.5253, 35.1939) -> (54.5253, 35.1558) centre (54.5253, 35.1748) ccw
  arc A109 (54.5253, 35.6116) -> (54.5253, 35.5735) centre (54.5253, 35.5926) ccw
  line L29 (54.5253, 35.1748) -> (54.3165, 35.1748)
  arc A110 (54.3165, 35.1939) -> (54.3165, 35.1558) centre (54.3165, 35.1748) ccw
  arc A111 (54.5253, 35.1558) -> (54.5253, 35.1939) centre (54.5253, 35.1748) ccw
  arc A112 (55.174, 27.6146) -> (55.174, 43.6146) centre (55.174, 35.6146) ccw
  arc A113 (55.174, 43.6146) -> (55.174, 27.6146) centre (55.174, 35.6146) ccw
  arc A114 (55.174, 29.0954) -> (55.174, 42.1338) centre (55.174, 35.6146) ccw
  arc A115 (55.174, 42.1338) -> (55.174, 29.0954) centre (55.174, 35.6146) ccw
  arc A116 (55.174, 26.1146) -> (55.174, 45.1146) centre (55.174, 35.6146) ccw
  arc A117 (55.174, 45.1146) -> (55.174, 26.1146) centre (55.174, 35.6146) ccw
  arc A118 (10.7101, 2.5843) -> (10.7101, 2.6859) centre (10.7101, 2.6351) ccw
  arc A119 (79.1431, 5.5907) -> (77.1431, 5.5907) centre (78.1431, 5.5907) ccw
  arc A120 (79.1114, 5.5907) -> (79.1749, 5.5907) centre (79.1431, 5.5907) ccw
  arc A121 (77.1114, 5.5907) -> (77.1749, 5.5907) centre (77.1431, 5.5907) ccw
  line L30 (83.1812, 11.8597) -> (83.4423, 12.0686)
  arc A122 (83.4542, 12.0537) -> (83.4304, 12.0834) centre (83.4423, 12.0686) ccw
  arc A123 (83.1693, 11.8746) -> (83.1931, 11.8448) centre (83.1812, 11.8597) ccw
  line L31 (83.4423, 12.0686) -> (83.4423, 11.1288)
  arc A124 (83.4232, 11.1288) -> (83.4613, 11.1288) centre (83.4423, 11.1288) ccw
  arc A125 (83.4613, 12.0686) -> (83.4232, 12.0686) centre (83.4423, 12.0686) ccw
  line L32 (83.1812, 11.1288) -> (83.7033, 11.1288)
  arc A126 (83.7033, 11.1097) -> (83.7033, 11.1478) centre (83.7033, 11.1288) ccw
  arc A127 (83.1812, 11.1478) -> (83.1812, 11.1097) centre (83.1812, 11.1288) ccw
  arc A128 (80.7033, 16.8336) -> (80.4684, 17.0686) centre (80.4683, 16.8336) ccw
  arc A129 (80.6843, 16.8336) -> (80.7224, 16.8336) centre (80.7034, 16.8336) ccw
  arc A130 (80.4684, 17.0876) -> (80.4684, 17.0495) centre (80.4684, 17.0686) ccw
  arc A131 (80.4684, 17.0686) -> (80.1812, 16.8597) centre (80.4684, 16.7667) ccw
  arc A132 (80.4684, 17.0495) -> (80.4684, 17.0876) centre (80.4684, 17.0686) ccw
  arc A133 (80.1631, 16.8656) -> (80.1993, 16.8538) centre (80.1812, 16.8597) ccw
  arc A134 (80.625, 16.6509) -> (80.7033, 16.8336) centre (80.4509, 16.8336) ccw
  arc A135 (2.5931, 2.6859) -> (2.5931, 2.5843) centre (2.5931, 2.6351) ccw
  arc A136 (80.7224, 16.8336) -> (80.6843, 16.8336) centre (80.7034, 16.8336) ccw
  line L33 (80.625, 16.6509) -> (80.1812, 16.1288)
  arc A137 (80.1667, 16.1411) -> (80.1957, 16.1164) centre (80.1812, 16.1288) ccw
  arc A138 (80.6395, 16.6385) -> (80.6105, 16.6632) centre (80.625, 16.6508) ccw
  line L34 (80.1812, 16.1288) -> (80.7033, 16.1288)
  arc A139 (80.7033, 16.1097) -> (80.7033, 16.1478) centre (80.7033, 16.1288) ccw
  arc A140 (80.1812, 16.1478) -> (80.1812, 16.1097) centre (80.1812, 16.1288) ccw
  line L35 (77.1812, 11.1288) -> (77.4423, 11.1288)
  arc A141 (77.4423, 11.1097) -> (77.4423, 11.1478) centre (77.4423, 11.1288) ccw
  arc A142 (77.1812, 11.1478) -> (77.1812, 11.1097) centre (77.1812, 11.1288) ccw
  arc A143 (77.4423, 11.1288) -> (77.4423, 11.6509) centre (77.4423, 11.3898) ccw
  arc A144 (77.4423, 11.1478) -> (77.4423, 11.1097) centre (77.4423, 11.1288) ccw
  arc A145 (77.4423, 11.6699) -> (77.4423, 11.6318) centre (77.4423, 11.6509) ccw
  line L36 (77.1812, 12.0686) -> (77.4945, 12.0686)
  arc A146 (77.4945, 12.0495) -> (77.4945, 12.0876) centre (77.4945, 12.0686) ccw
  arc A147 (77.1812, 12.0876) -> (77.1812, 12.0495) centre (77.1812, 12.0686) ccw
  arc A148 (77.4945, 11.6509) -> (77.4945, 12.0686) centre (77.4945, 11.8598) ccw
  arc A149 (77.4945, 11.6699) -> (77.4945, 11.6318) centre (77.4945, 11.6509) ccw
  arc A150 (77.4945, 12.0876) -> (77.4945, 12.0495) centre (77.4945, 12.0686) ccw
  line L37 (77.4945, 11.6509) -> (77.2856, 11.6509)
  arc A151 (77.2856, 11.6699) -> (77.2856, 11.6318) centre (77.2856, 11.6509) ccw
  arc A152 (77.4945, 11.6318) -> (77.4945, 11.6699) centre (77.4945, 11.6509) ccw
  arc A153 (78.1431, 4.0907) -> (78.1431, 20.0907) centre (78.1431, 12.0907) ccw
  arc A154 (78.1431, 20.0907) -> (78.1431, 4.0907) centre (78.1431, 12.0907) ccw
  arc A155 (78.1431, 5.5715) -> (78.1431, 18.6099) centre (78.1431, 12.0907) ccw
  arc A156 (78.1431, 18.6099) -> (78.1431, 5.5715) centre (78.1431, 12.0907) ccw
  arc A157 (78.1431, 2.5907) -> (78.1431, 21.5907) centre (78.1431, 12.0907) ccw
  arc A158 (78.1431, 21.5907) -> (78.1431, 2.5907) centre (78.1431, 12.0907) ccw
  line L38 (10.7101, 2.6351) -> (2.5931, 2.6351)
  arc A159 (34.6686, 29.1146) -> (32.6686, 29.1146) centre (33.6686, 29.1146) ccw
  arc A160 (34.6369, 29.1146) -> (34.7004, 29.1146) centre (34.6686, 29.1146) ccw
  arc A161 (32.6369, 29.1146) -> (32.7004, 29.1146) centre (32.6686, 29.1146) ccw
  line L39 (38.7067, 35.3837) -> (38.9678, 35.5925)
  arc A162 (38.9797, 35.5776) -> (38.9559, 35.6074) centre (38.9678, 35.5925) ccw
  arc A163 (38.6948, 35.3985) -> (38.7186, 35.3688) centre (38.7067, 35.3837) ccw
  line L40 (38.9678, 35.5925) -> (38.9678, 34.6527)
  arc A164 (38.9487, 34.6527) -> (38.9868, 34.6527) centre (38.9678, 34.6527) ccw
  arc A165 (38.9868, 35.5925) -> (38.9487, 35.5925) centre (38.9678, 35.5925) ccw
  line L41 (38.7067, 34.6527) -> (39.2288, 34.6527)
  arc A166 (39.2288, 34.6337) -> (39.2288, 34.6718) centre (39.2288, 34.6527) ccw
  arc A167 (38.7067, 34.6718) -> (38.7067, 34.6337) centre (38.7067, 34.6527) ccw
  arc A168 (36.2288, 40.3576) -> (35.9939, 40.5925) centre (35.9939, 40.3576) ccw
  arc A169 (36.2098, 40.3576) -> (36.2479, 40.3576) centre (36.2289, 40.3576) ccw
  arc A170 (35.9939, 40.6116) -> (35.9939, 40.5735) centre (35.9939, 40.5926) ccw
  arc A171 (35.9939, 40.5925) -> (35.7067, 40.3837) centre (35.9938, 40.2907) ccw
  arc A172 (35.9939, 40.5735) -> (35.9939, 40.6116) centre (35.9939, 40.5926) ccw
  arc A173 (35.6886, 40.3895) -> (35.7248, 40.3778) centre (35.7067, 40.3837) ccw
  arc A174 (36.1505, 40.1748) -> (36.2288, 40.3576) centre (35.9763, 40.3576) ccw
  arc A175 (36.1374, 40.1886) -> (36.1637, 40.161) centre (36.1505, 40.1748) ccw
  arc A176 (36.2479, 40.3576) -> (36.2098, 40.3576) centre (36.2289, 40.3576) ccw
  line L42 (36.1505, 40.1748) -> (35.7067, 39.6527)
  arc A177 (35.6922, 39.665) -> (35.7212, 39.6404) centre (35.7067, 39.6527) ccw
  arc A178 (36.165, 40.1625) -> (36.136, 40.1872) centre (36.1505, 40.1748) ccw
  line L43 (35.7067, 39.6527) -> (36.2288, 39.6527)
  arc A179 (36.2288, 39.6337) -> (36.2288, 39.6718) centre (36.2288, 39.6527) ccw
  arc A180 (35.7067, 39.6718) -> (35.7067, 39.6337) centre (35.7067, 39.6527) ccw
  line L44 (32.7067, 34.6527) -> (32.9678, 34.6527)
  arc A181 (32.9678, 34.6337) -> (32.9678, 34.6718) centre (32.9678, 34.6527) ccw
  arc A182 (32.7067, 34.6718) -> (32.7067, 34.6337) centre (32.7067, 34.6527) ccw
  arc A183 (32.9678, 34.6527) -> (32.9678, 35.1748) centre (32.9678, 34.9138) ccw
  arc A184 (32.9678, 34.6718) -> (32.9678, 34.6337) centre (32.9678, 34.6527) ccw
  arc A185 (32.9678, 35.1939) -> (32.9678, 35.1558) centre (32.9678, 35.1748) ccw
  line L45 (32.7067, 35.5925) -> (33.02, 35.5925)
  arc A186 (33.02, 35.5735) -> (33.02, 35.6116) centre (33.02, 35.5926) ccw
  arc A187 (32.7067, 35.6116) -> (32.7067, 35.5735) centre (32.7067, 35.5926) ccw
  arc A188 (33.02, 35.1748) -> (33.02, 35.5925) centre (33.02, 35.3837) ccw
  arc A189 (33.02, 35.1939) -> (33.02, 35.1558) centre (33.02, 35.1748) ccw
  arc A190 (33.02, 35.6116) -> (33.02, 35.5735) centre (33.02, 35.5926) ccw
  line L46 (33.02, 35.1748) -> (32.8112, 35.1748)
  arc A191 (32.8112, 35.1939) -> (32.8112, 35.1558) centre (32.8112, 35.1748) ccw
  arc A192 (33.02, 35.1558) -> (33.02, 35.1939) centre (33.02, 35.1748) ccw
  arc A193 (33.6686, 27.6146) -> (33.6686, 43.6146) centre (33.6686, 35.6146) ccw
  arc A194 (33.6686, 43.6146) -> (33.6686, 27.6146) centre (33.6686, 35.6146) ccw
  arc A195 (33.6686, 29.0954) -> (33.6686, 42.1338) centre (33.6686, 35.6146) ccw
  arc A196 (33.6686, 42.1338) -> (33.6686, 29.0954) centre (33.6686, 35.6146) ccw
  arc A197 (33.6686, 26.1146) -> (33.6686, 45.1146) centre (33.6686, 35.6146) ccw
  arc A198 (33.6686, 45.1146) -> (33.6686, 26.1146) centre (33.6686, 35.6146) ccw
  arc A199 (14.4761, 2.5843) -> (14.4761, 2.6859) centre (14.4761, 2.6351) ccw
  arc A200 (13.1633, 29.1146) -> (11.1633, 29.1146) centre (12.1633, 29.1146) ccw
  arc A201 (13.1315, 29.1146) -> (13.195, 29.1146) centre (13.1633, 29.1146) ccw
  arc A202 (11.1315, 29.1146) -> (11.195, 29.1146) centre (11.1633, 29.1146) ccw
  line L47 (17.2014, 35.3837) -> (17.4625, 35.5925)
  arc A203 (17.4744, 35.5776) -> (17.4505, 35.6074) centre (17.4625, 35.5925) ccw
  arc A204 (17.1895, 35.3985) -> (17.2133, 35.3688) centre (17.2014, 35.3837) ccw
  line L48 (17.4625, 35.5925) -> (17.4625, 34.6527)
  arc A205 (17.4434, 34.6527) -> (17.4815, 34.6527) centre (17.4625, 34.6527) ccw
  arc A206 (17.4815, 35.5925) -> (17.4434, 35.5925) centre (17.4625, 35.5925) ccw
  line L49 (17.2014, 34.6527) -> (17.7235, 34.6527)
  arc A207 (17.7235, 34.6337) -> (17.7235, 34.6718) centre (17.7235, 34.6527) ccw
  arc A208 (17.2014, 34.6718) -> (17.2014, 34.6337) centre (17.2014, 34.6527) ccw
  arc A209 (14.7235, 40.3576) -> (14.4886, 40.5925) centre (14.4886, 40.3576) ccw
  arc A210 (14.7045, 40.3576) -> (14.7426, 40.3576) centre (14.7236, 40.3576) ccw
  arc A211 (14.4886, 40.6116) -> (14.4886, 40.5735) centre (14.4886, 40.5926) ccw
  arc A212 (14.4886, 40.5925) -> (14.2014, 40.3837) centre (14.4885, 40.2907) ccw
  arc A213 (14.4886, 40.5735) -> (14.4886, 40.6116) centre (14.4886, 40.5926) ccw
  arc A214 (14.1833, 40.3895) -> (14.2195, 40.3778) centre (14.2014, 40.3837) ccw
  arc A215 (14.6452, 40.1748) -> (14.7235, 40.3576) centre (14.471, 40.3576) ccw
  arc A216 (14.6321, 40.1886) -> (14.6583, 40.161) centre (14.6452, 40.1748) ccw
  arc A217 (14.7426, 40.3576) -> (14.7045, 40.3576) centre (14.7236, 40.3576) ccw
  line L50 (14.6452, 40.1748) -> (14.2014, 39.6527)
  arc A218 (14.1869, 39.665) -> (14.2159, 39.6404) centre (14.2014, 39.6527) ccw
  arc A219 (14.6597, 40.1625) -> (14.6307, 40.1872) centre (14.6452, 40.1748) ccw
  line L51 (14.2014, 39.6527) -> (14.7235, 39.6527)
  arc A220 (14.7235, 39.6337) -> (14.7235, 39.6718) centre (14.7235, 39.6527) ccw
  arc A221 (14.2014, 39.6718) -> (14.2014, 39.6337) centre (14.2014, 39.6527) ccw
  line L52 (11.2014, 34.6527) -> (11.4625, 34.6527)
  arc A222 (11.4625, 34.6337) -> (11.4625, 34.6718) centre (11.4625, 34.6527) ccw
  arc A223 (11.2014, 34.6718) -> (11.2014, 34.6337) centre (11.2014, 34.6527) ccw
  arc A224 (11.4625, 34.6527) -> (11.4625, 35.1748) centre (11.4625, 34.9138) ccw
  arc A225 (11.4625, 34.6718) -> (11.4625, 34.6337) centre (11.4625, 34.6527) ccw
  arc A226 (11.4625, 35.1939) -> (11.4625, 35.1558) centre (11.4625, 35.1748) ccw
  line L53 (11.2014, 35.5925) -> (11.5147, 35.5925)
  arc A227 (11.5147, 35.5735) -> (11.5147, 35.6116) centre (11.5147, 35.5926) ccw
  arc A228 (11.2014, 35.6116) -> (11.2014, 35.5735) centre (11.2014, 35.5926) ccw
  arc A229 (11.5147, 35.1748) -> (11.5147, 35.5925) centre (11.5147, 35.3837) ccw
  arc A230 (11.5147, 35.1939) -> (11.5147, 35.1558) centre (11.5147, 35.1748) ccw
  arc A231 (11.5147, 35.6116) -> (11.5147, 35.5735) centre (11.5147, 35.5926) ccw
  line L54 (11.5147, 35.1748) -> (11.3058, 35.1748)
  arc A232 (11.3058, 35.1939) -> (11.3058, 35.1558) centre (11.3058, 35.1748) ccw
  arc A233 (11.5147, 35.1558) -> (11.5147, 35.1939) centre (11.5147, 35.1748) ccw
  arc A234 (12.1633, 27.6146) -> (12.1633, 43.6146) centre (12.1633, 35.6146) ccw
  arc A235 (12.1633, 43.6146) -> (12.1633, 27.6146) centre (12.1633, 35.6146) ccw
  arc A236 (12.1633, 29.0954) -> (12.1633, 42.1338) centre (12.1633, 35.6146) ccw
  arc A237 (12.1633, 42.1338) -> (12.1633, 29.0954) centre (12.1633, 35.6146) ccw
  arc A238 (12.1633, 26.1146) -> (12.1633, 45.1146) centre (12.1633, 35.6146) ccw
  arc A239 (12.1633, 45.1146) -> (12.1633, 26.1146) centre (12.1633, 35.6146) ccw
  arc A240 (76.2847, 35.1558) -> (76.2847, 35.1939) centre (76.2847, 35.1748) ccw
  arc A241 (96.25, 17.63) -> (94.25, 17.63) centre (95.25, 17.63) ccw
  arc A242 (96.2182, 17.63) -> (96.2818, 17.63) centre (96.25, 17.63) ccw
  arc A243 (94.2182, 17.63) -> (94.2818, 17.63) centre (94.25, 17.63) ccw
  line L55 (100.2881, 23.8991) -> (100.5492, 24.1079)
  arc A244 (100.5611, 24.093) -> (100.5373, 24.1228) centre (100.5492, 24.1079) ccw
  arc A245 (100.2762, 23.9139) -> (100.3, 23.8842) centre (100.2881, 23.8991) ccw
  line L56 (100.5492, 24.1079) -> (100.5492, 23.1681)
  arc A246 (100.5301, 23.1681) -> (100.5682, 23.1681) centre (100.5492, 23.1681) ccw
  arc A247 (100.5682, 24.1079) -> (100.5301, 24.1079) centre (100.5492, 24.1079) ccw
  line L57 (100.2881, 23.1681) -> (100.8102, 23.1681)
  arc A248 (100.8102, 23.1491) -> (100.8102, 23.1872) centre (100.8102, 23.1682) ccw
  arc A249 (100.2881, 23.1872) -> (100.2881, 23.1491) centre (100.2881, 23.1682) ccw
  arc A250 (97.8102, 28.873) -> (97.5753, 29.1079) centre (97.5753, 28.873) ccw
  arc A251 (97.7912, 28.873) -> (97.8293, 28.873) centre (97.8102, 28.873) ccw
  arc A252 (97.5753, 29.127) -> (97.5753, 29.0889) centre (97.5753, 29.108) ccw
  arc A253 (97.5753, 29.1079) -> (97.2881, 28.8991) centre (97.5752, 28.8061) ccw
  arc A254 (97.5753, 29.0889) -> (97.5753, 29.1269) centre (97.5753, 29.1079) ccw
  arc A255 (97.27, 28.9049) -> (97.3062, 28.8932) centre (97.2881, 28.8991) ccw
  arc A256 (97.7319, 28.6902) -> (97.8102, 28.873) centre (97.5577, 28.873) ccw
  arc A257 (97.7188, 28.704) -> (97.745, 28.6764) centre (97.7319, 28.6902) ccw
  arc A258 (97.8293, 28.8729) -> (97.7912, 28.873) centre (97.8102, 28.873) ccw
  line L58 (97.7319, 28.6902) -> (97.2881, 28.1681)
  arc A259 (97.2736, 28.1804) -> (97.3026, 28.1558) centre (97.2881, 28.1681) ccw
  arc A260 (97.7464, 28.6779) -> (97.7174, 28.7025) centre (97.7319, 28.6902) ccw
  line L59 (97.2881, 28.1681) -> (97.8102, 28.1681)
  arc A261 (97.8102, 28.1491) -> (97.8102, 28.1872) centre (97.8102, 28.1682) ccw
  arc A262 (97.2881, 28.1872) -> (97.2881, 28.1491) centre (97.2881, 28.1682) ccw
  line L60 (94.2881, 23.1681) -> (94.5492, 23.1681)
  arc A263 (94.5492, 23.1491) -> (94.5492, 23.1872) centre (94.5492, 23.1682) ccw
  arc A264 (94.2881, 23.1872) -> (94.2881, 23.1491) centre (94.2881, 23.1682) ccw
  arc A265 (94.5492, 23.1681) -> (94.5492, 23.6902) centre (94.5492, 23.4291) ccw
  arc A266 (94.5492, 23.1872) -> (94.5492, 23.1491) centre (94.5492, 23.1682) ccw
  arc A267 (94.5492, 23.7093) -> (94.5492, 23.6712) centre (94.5492, 23.6903) ccw
  line L61 (94.2881, 24.1079) -> (94.6014, 24.1079)
  arc A268 (94.6014, 24.0889) -> (94.6014, 24.127) centre (94.6014, 24.108) ccw
  arc A269 (94.2881, 24.127) -> (94.2881, 24.0889) centre (94.2881, 24.108) ccw
  arc A270 (94.6014, 23.6902) -> (94.6014, 24.1079) centre (94.6014, 23.8991) ccw
  arc A271 (94.6014, 23.7093) -> (94.6014, 23.6712) centre (94.6014, 23.6903) ccw
  arc A272 (94.6014, 24.127) -> (94.6014, 24.0889) centre (94.6014, 24.108) ccw
  line L62 (94.6014, 23.6902) -> (94.3925, 23.6902)
  arc A273 (94.3925, 23.7093) -> (94.3925, 23.6712) centre (94.3925, 23.6903) ccw
  arc A274 (94.6014, 23.6712) -> (94.6014, 23.7093) centre (94.6014, 23.6903) ccw
  arc A275 (95.25, 16.13) -> (95.25, 32.13) centre (95.25, 24.13) ccw
  arc A276 (95.25, 32.13) -> (95.25, 16.13) centre (95.25, 24.13) ccw
  arc A277 (95.25, 17.6108) -> (95.25, 30.6492) centre (95.25, 24.13) ccw
  arc A278 (95.25, 30.6492) -> (95.25, 17.6108) centre (95.25, 24.13) ccw
  arc A279 (95.25, 14.63) -> (95.25, 33.63) centre (95.25, 24.13) ccw
  arc A280 (95.25, 33.63) -> (95.25, 14.63) centre (95.25, 24.13) ccw
  arc A281 (76.2324, 34.6337) -> (76.2324, 34.6718) centre (76.2324, 34.6527) ccw
  line L63 (75.9714, 34.6527) -> (76.2324, 34.6527)
  arc A282 (78.9714, 39.6718) -> (78.9714, 39.6337) centre (78.9714, 39.6527) ccw
  arc A283 (79.4935, 39.6337) -> (79.4935, 39.6718) centre (79.4935, 39.6527) ccw
  line L64 (78.9714, 39.6527) -> (79.4935, 39.6527)
  arc A284 (79.4297, 40.1625) -> (79.4007, 40.1872) centre (79.4152, 40.1748) ccw
  arc A285 (78.9569, 39.665) -> (78.9859, 39.6404) centre (78.9714, 39.6527) ccw
  line L65 (79.4152, 40.1748) -> (78.9714, 39.6527)
  arc A286 (79.5125, 40.3576) -> (79.4745, 40.3576) centre (79.4935, 40.3576) ccw
  arc A287 (79.402, 40.1886) -> (79.4283, 40.161) centre (79.4151, 40.1748) ccw
  arc A288 (79.4152, 40.1748) -> (79.4935, 40.3576) centre (79.241, 40.3576) ccw
  arc A289 (78.9533, 40.3895) -> (78.9895, 40.3778) centre (78.9714, 40.3837) ccw
  arc A290 (79.2586, 40.5735) -> (79.2585, 40.6116) centre (79.2585, 40.5926) ccw
  arc A291 (79.2585, 40.5925) -> (78.9714, 40.3837) centre (79.2585, 40.2907) ccw
  arc A292 (79.2585, 40.6116) -> (79.2585, 40.5735) centre (79.2585, 40.5926) ccw
  arc A293 (79.4745, 40.3576) -> (79.5125, 40.3576) centre (79.4935, 40.3576) ccw
  arc A294 (79.4935, 40.3576) -> (79.2585, 40.5925) centre (79.2585, 40.3575) ccw
  arc A295 (81.9714, 34.6718) -> (81.9714, 34.6337) centre (81.9714, 34.6527) ccw
  arc A296 (82.4935, 34.6337) -> (82.4935, 34.6718) centre (82.4935, 34.6527) ccw
  line L66 (81.9714, 34.6527) -> (82.4935, 34.6527)
  arc A297 (82.2515, 35.5925) -> (82.2134, 35.5925) centre (82.2325, 35.5925) ccw
  arc A298 (82.2134, 34.6527) -> (82.2515, 34.6527) centre (82.2325, 34.6527) ccw
  line L67 (82.2324, 35.5925) -> (82.2324, 34.6527)
  arc A299 (81.9595, 35.3985) -> (81.9833, 35.3688) centre (81.9714, 35.3837) ccw
  arc A300 (82.2443, 35.5776) -> (82.2205, 35.6074) centre (82.2324, 35.5925) ccw
  line L68 (81.9714, 35.3837) -> (82.2324, 35.5925)
  arc A301 (75.9015, 29.1146) -> (75.965, 29.1146) centre (75.9333, 29.1146) ccw
  arc A302 (77.9015, 29.1146) -> (77.965, 29.1146) centre (77.9333, 29.1146) ccw
  arc A303 (77.9333, 29.1146) -> (75.9333, 29.1146) centre (76.9333, 29.1146) ccw
  arc A304 (26.7722, 17.1013) -> (26.8218, 17.0617) centre (26.797, 17.0815) ccw
  arc A305 (27.3298, 17.6967) -> (27.2802, 17.7363) centre (27.305, 17.7165) ccw
  line L69 (26.797, 17.0815) -> (27.305, 17.7165)
  arc A306 (27.3033, 16.976) -> (27.2432, 16.9965) centre (27.2733, 16.9862) ccw
  arc A307 (27.051, 16.8592) -> (27.051, 16.7958) centre (27.051, 16.8275) ccw
  arc A308 (27.051, 16.8275) -> (27.2733, 16.9863) centre (27.051, 17.0625) ccw
  arc A309 (27.4002, 17.399) -> (27.3368, 17.399) centre (27.3685, 17.399) ccw
  arc A310 (27.2447, 17.0002) -> (27.3018, 16.9723) centre (27.2733, 16.9862) ccw
  arc A311 (27.2733, 16.9863) -> (27.3685, 17.399) centre (26.4268, 17.3989) ccw
  arc A312 (27.051, 16.7958) -> (27.051, 16.8592) centre (27.051, 16.8275) ccw
  arc A313 (26.8588, 16.9965) -> (26.7987, 16.976) centre (26.8287, 16.9862) ccw
  arc A314 (26.8288, 16.9863) -> (27.051, 16.8275) centre (27.051, 17.0624) ccw
  arc A315 (26.8002, 16.9723) -> (26.8573, 17.0002) centre (26.8287, 16.9862) ccw
  arc A316 (26.7653, 17.399) -> (26.7018, 17.399) centre (26.7336, 17.399) ccw
  arc A317 (26.7335, 17.399) -> (26.8288, 16.9863) centre (27.6752, 17.3991) ccw
  arc A318 (27.3018, 17.8257) -> (27.2447, 17.7978) centre (27.2733, 17.8118) ccw
  arc A319 (27.3368, 17.399) -> (27.4002, 17.399) centre (27.3685, 17.399) ccw